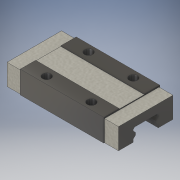
# Autodesk Inventor part: mgn9h_carriage
Saved by Autodesk Inventor 2017 (Build 210142000, 142)
## iProperties
Created: 2016-06-03
Part Number: mgn9h_carriage
Material: Generic
Document SubType Name: Modeling
Designer: brent
Density: 1 g/cm^3
Appearance: Steel Galvanized
Author: brent
Autodesk Inventor part; units mm, degrees
ref_plane "YZ Plane" through (0, 0, 0) normal (1, 0, 0) x (0, 1, 0)
ref_plane "XZ Plane" through (0, 0, 0) normal (0, 1, 0) x (-1, 0, 0)
sketch "Sketch1" plane through (0, 0, 0) normal (1, 0, 0) x (0, 1, 0)
  line L0 (0, 0) -> (2, 0)
  line L1 (6.5, 0) -> (6.5, -9)
  line L2 (6.5, -9) -> (2, -9)
  line L3 (0, -9) -> (0, 0)
  line L4 (10, 5.5) -> (2, 5.5)
  line L5 (2, 5.5) -> (2, 0)
  line L6 (2, -14.5) -> (10, -14.5)
  line L7 (10, -14.5) -> (10, 5.5)
  line L8 (10, -4.5) -> (6.5, -4.5)
  line L9 (2, 0) -> (6.5, 0)
  line L10 (2, 0) -> (2, -14.5)
  line L11 (2, -9) -> (0, -9)
  dimension "d0" = 6.5
  dimension "d1" = 9
  dimension "d3" = 10
  dimension "d4" = 20
  dimension "d5" = 2
  constraints: 24 end point, 8 parallel, 4 horizontal, 4 perpendicular, 2 midpoint, 1 point on line
  measures "d0" distance of L1.end L3.start
  measures "d1" distance of L1.start L1.end
  measures "d3" distance between parallel lines of L3 L7
  measures "d4" distance of L6.end L4.start
  measures "d5" distance between parallel lines of L3 L5
extrude "Extrusion1" add sketch "Sketch1" along normal blind 39.9 contours L5 L4 L7 L8 L1 L9 | L2 L1 L8 L7 L6 L10
sketch "Sketch2" plane through (39.9, 0, 0) normal (1, 0, 0) x (0, 0, -1)
  line L0 (0, 6.5) -> (9, 6.5) projected
  line L1 (9, 6.5) -> (9, 2) projected
  line L2 (9, 2) -> (14.5, 2) projected
  line L3 (14.5, 2) -> (14.5, 10) projected
  line L4 (14.5, 10) -> (-5.5, 10) projected
  line L5 (-5.5, 10) -> (-5.5, 2) projected
  line L6 (-5.5, 2) -> (0, 2) projected
  line L7 (0, 2) -> (0, 6.5) projected
  line L8 (0, 5.5) -> (1.25, 4.25)
  line L9 (1.25, 4.25) -> (0, 3)
  line L10 (9, 5.5) -> (7.75, 4.25)
  line L11 (7.75, 4.25) -> (9, 3)
  line L12 (9, 6.5) -> (9, 2) projected
  line L13 (9, 5.5) -> (0, 5.5)
  line L14 (0, 3) -> (9, 3)
  point P0 (0, 0)
  dimension "d8" = 90
  dimension "d9" = 45
  dimension "d10" = 3.5
  dimension "d11" = 1
  dimension "d12" = 45
  constraints: 12 end point, 4 point on line, 2 horizontal, 1 perpendicular
  measures "d8" angle of L9 L8
  measures "d9" angle of L7 L8
  measures "d10" distance from line of L0 L9.end
  measures "d11" distance from line of L0 L8.start
  measures "d12" angle of L1 L10
extrude "Extrusion2" add sketch "Sketch2" against normal up to surface (39.9 mm away) contours L8 L9 L7 | L1 L11 L10
chamfer "Chamfer1" distance 0.5 angle 45 4 edges at (19.95, 6.5, -9) (19.95, 6.5, 0) (19.95, 4.25, -1.25) (19.95, 4.25, -7.75)
sketch "Sketch3" plane through (0, 10, 5.5) normal (0, 1, 0) x (1, 0, 0)
  line L0 (0, 20) -> (0, 0) projected
  line L1 (0, 0) -> (39.9, 0) projected
  line L2 (39.9, 20) -> (39.9, 0) projected
  line L3 (0, 20) -> (39.9, 20) projected
  line L4 (0, 0) -> (39.9, 20) construction
  line L5 (27.95, 2.5) -> (11.95, 2.5)
  line L6 (11.95, 2.5) -> (11.95, 17.5)
  line L7 (11.95, 17.5) -> (27.95, 17.5)
  line L8 (27.95, 17.5) -> (27.95, 2.5)
  line L9 (27.95, 2.5) -> (11.95, 17.5) construction
  line L10 (11.95, 2.5) -> (27.95, 17.5) construction
  circle A0 centre (11.95, 17.5) radius 1.5
  circle A1 centre (27.95, 17.5) radius 1.5
  circle A2 centre (27.95, 2.5) radius 1.5
  circle A3 centre (11.95, 2.5) radius 1.5
  point P0 (0, 5.5)
  point P1 (19.95, 10)
  dimension "d18" = 16
  dimension "d19" = 15
  dimension "d20" = 3
  dimension "d21" = 3
  dimension "d22" = 3
  dimension "d23" = 3
  constraints: 14 end point, 4 centre point, 4 coincident, 3 midpoint, 2 parallel, 1 horizontal, 1 perpendicular
  measures "d18" distance of L6.end L7.end
  measures "d19" distance of L5.end L6.end
  measures "d20" diameter of A0
  measures "d21" diameter of A1
  measures "d22" diameter of A2
  measures "d23" diameter of A3
extrude "Extrusion3" cut sketch "Sketch3" against normal blind 3 contours A3 L6 L5 | L5 L6 A3 | A2 L8 L5 | L5 L8 A2 | A0 L7 L6 | L6 L7 A0 | A1 L7 L8 | L8 L7 A1
sketch "Sketch4" plane through (0, 10, 5.5) normal (0, 1, 0) x (1, 0, 0)
  circle A0 centre (11.95, 2.5) radius 1.5 projected
  circle A1 centre (27.95, 17.5) radius 1.5 projected
  circle A2 centre (11.95, 17.5) radius 1.5 projected
  circle A3 centre (27.95, 2.5) radius 1.5 projected
  line L0 (0, 20) -> (0, 0) projected
  line L1 (0, 0) -> (39.9, 0) projected
  line L2 (39.9, 20) -> (39.9, 0) projected
  line L3 (0, 20) -> (39.9, 20) projected
  line L4 (39.9, 20) -> (39.9, 0) projected
  line L5 (0, 5.5) -> (39.9, 5.5)
  line L6 (39.9, 5.5) -> (39.9, 14.5)
  line L7 (39.9, 14.5) -> (0, 14.5)
  line L8 (0, 14.5) -> (0, 5.5)
  line L9 (0, 14.5) -> (39.9, 14.5) projected
  constraints: 8 end point, 2 parallel, 2 point on line, 1 horizontal, 1 perpendicular
extrude "Extrusion4" cut sketch "Sketch4" against normal blind 0.2 contours L7 L2 L5 L0
sketch "Sketch5" plane through (39.9, 0, 0) normal (1, 0, 0) x (0, 0, -1)
  line L0 (0, 9.8) -> (0, 10) projected
  line L1 (0, 10) -> (-5.5, 10) construction
  line L2 (-5.5, 10) -> (-5.5, 2) projected
  line L3 (-5.5, 2) -> (0, 2) projected
  line L4 (0, 2) -> (0, 3) projected
  line L5 (0, 3) -> (0.8964, 3.8964) projected
  line L6 (0.8964, 4.6036) -> (0.8964, 3.8964) projected
  line L7 (0.8964, 4.6036) -> (0, 5.5) projected
  line L8 (0, 5.5) -> (0, 6) construction
  line L9 (0.5, 6.5) -> (0, 6) construction
  line L10 (0.5, 6.5) -> (8.5, 6.5) projected
  line L11 (9, 6) -> (8.5, 6.5) projected
  line L12 (9, 6) -> (9, 5.5) projected
  line L13 (9, 5.5) -> (8.1036, 4.6036) construction
  line L14 (8.1036, 3.8964) -> (8.1036, 4.6036) construction
  line L15 (8.1036, 3.8964) -> (9, 3) construction
  line L16 (9, 3) -> (9, 2) projected
  line L17 (9, 2) -> (14.5, 2) projected
  line L18 (14.5, 2) -> (14.5, 10) projected
  line L19 (14.5, 10) -> (9, 10) projected
  line L20 (9, 10) -> (9, 9.8) projected
  line L21 (9, 9.8) -> (0, 9.8) projected
  line L22 (-5.25, 9.5) -> (14.25, 9.5)
  line L23 (14.25, 9.5) -> (14.25, 2)
  line L24 (14.25, 2) -> (-5.25, 2)
  line L25 (-5.25, 2) -> (-5.25, 9.5)
  circle A0 centre (4.5, 2) radius 50
  point P0 (0, 0)
  dimension "d28" = 0.25
  dimension "d29" = 0.25
  dimension "d30" = 0.5
  dimension "d31" = 100
  constraints: 8 end point, 2 parallel, 1 centre point, 1 horizontal, 1 midpoint, 1 perpendicular, 1 point on line
  measures "d28" distance between parallel lines of L2 L25
  measures "d29" distance between parallel lines of L18 L23
  measures "d30" distance between parallel lines of L1 L22
  measures "d31" diameter of A0
extrude "Extrusion5" cut sketch "Sketch5" against normal blind 5
ref_plane "Work Plane1" through (19.95, 0, 0) normal (1, 0, 0) x (0, 0, -1)
mirror "Mirror1" about plane through (19.95, 0, 0) normal (1, 0, 0) of "Extrusion5"
body "Solid1"
